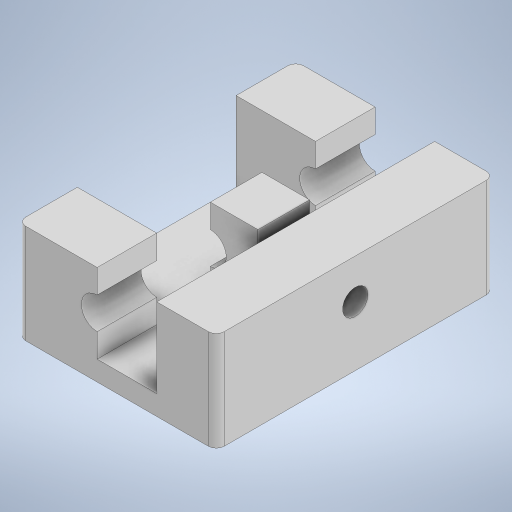
# Autodesk Inventor part: RodBender
Saved by Autodesk Inventor 2023 (Build 270158000, 158)
## iProperties
Created: 2024-04-01
Part Number: RodBender
Material: Generic
Document SubType Name: Modeling
Designer: incep
Density: 1 g/cm^3
Appearance: Default
Author: incep
## iProperties of the stored document RodBender_3DPrint.ipt
Created: 2024-04-01
Part Number: RodBender_3DPrint
Material: Generic
Document SubType Name: Modeling
Designer: incep
Density: 1 g/cm^3
Appearance: Default
Author: incep
Autodesk Inventor part; units mm, degrees
ref_plane "YZ Plane" through (0, 0, 0) normal (1, 0, 0) x (0, 1, 0)
ref_plane "XZ Plane" through (0, 0, 0) normal (0, 1, 0) x (-1, 0, 0)
ref_plane "XY Plane" through (0, 0, 0) normal (0, 0, 1) x (1, 0, 0)
sketch "Sketch1" plane through (0, 0, 0) normal (0, 1, 0) x (-1, 0, 0)
  line L0 (25, -35) -> (-25, -35)
  line L1 (-25, -35) -> (-25, 35)
  line L2 (-25, 35) -> (25, 35)
  line L3 (25, 35) -> (25, -35)
  line L4 (25, -35) -> (5, -35)
  line L5 (5, -35) -> (5, 35)
  line L6 (5, 35) -> (25, 35)
  line L7 (25, 35) -> (25, -35)
  line L8 (-10, -35) -> (-25, -35)
  line L9 (-25, -35) -> (-25, 35)
  line L10 (-25, 35) -> (-10, 35)
  line L11 (-10, 35) -> (-10, -35)
  line L12 (5, 6.5) -> (-7, 6.5)
  line L13 (-7, 6.5) -> (-7, -6.5)
  line L14 (-7, -6.5) -> (5, -6.5)
  line L15 (5, -6.5) -> (5, 6.5)
  point P0 (0, 0)
  point P1 (-25, 0)
  point P2 (0, -35)
  point P3 (5, 0)
  point P4 (5, -35)
  point P5 (-10, -7.5)
  point P6 (5, -6.5)
  point P7 (5, 6.5)
  point P8 (-10, 7.5)
  dimension "d0" = 70
  dimension "d1" = 50
  dimension "d2" = 20
  dimension "d3" = 15
  dimension "d4" = 13
  dimension "d16" = 3
  constraints: 32 end point, 8 parallel, 4 horizontal, 4 midpoint, 4 perpendicular, 2 point on line, 1 collinear, 1 horizontal alignment, 1 vertical alignment
  measures "d0" distance of L2.end L0.start
  measures "d1" distance of L0.start L0.end
  measures "d2" distance between parallel lines of L5 L3
  measures "d3" distance between parallel lines of L1 L11
  measures "d4" distance between parallel lines of L14 L12
  measures "d16" distance between parallel lines of L11 L13
extrude "Extrusion1" add sketch "Sketch1" against normal blind 5
extrude "Extrusion2" add sketch "Sketch1" along normal blind 20 contours L0 L5 L2 L3 | L0 L1 L2 L11
extrude "Extrusion3" add sketch "Sketch1" along normal blind 20 separate body contours L14 L13 L12 L5
sketch "Sketch2" plane through (25, -5, -35) normal (0, 0, -1) x (-1, 0, 0)
  line L0 (30, 5) -> (30, 25) projected
  circle A0 centre (30, 15) radius 4
  point P0 (25, 5)
  dimension "d11" = 8
  constraints: 1 centre point, 1 midpoint
  measures "d11" diameter of A0
extrude "Extrusion4" cut sketch "Sketch2" against normal up to surface (70 mm away) bodies 1
extrude "Extrusion5" cut sketch "Sketch2" against normal up to surface (70 mm away) bodies 2
sketch "Sketch3" plane through (0, 20, 0) normal (0, 1, 0) x (1, 0, 0)
  line L0 (-25, -35) -> (-25, 35) projected
  line L1 (-5, -35) -> (-5, 35) projected
  line L2 (-25, 20) -> (-5, 20)
  line L3 (-5, 20) -> (-5, -20)
  line L4 (-5, -20) -> (-25, -20)
  line L5 (-25, -20) -> (-25, 20)
  point P0 (0, 0)
  point P1 (-25, 0)
  point P2 (-5, 20)
  dimension "d17" = 40
  constraints: 8 end point, 2 midpoint, 2 parallel, 2 point on line, 1 horizontal, 1 perpendicular
  measures "d17" distance between parallel lines of L4 L2
extrude "Extrusion6" cut sketch "Sketch3" against normal up to surface (20 mm away) bodies 1
sketch "Sketch4" plane through (25, -5, 35) normal (1, 0, 0) x (0, 0, -1)
  line L0 (35, 5) -> (35, 25) construction
  line L1 (28.5, 25) -> (41.5, 25) construction
  circle A0 centre (35, 15) radius 3.2
  dimension "d20" = 6.4
  constraints: 2 end point, 2 midpoint, 1 centre point
  measures "d20" diameter of A0
extrude "Extrusion7" cut sketch "Sketch4" against normal up to surface (15 mm away) bodies 1
fillet "Fillet1" radius 2 4 edges at (-25, 7.5, 35) (25, 7.5, 35) (-25, 7.5, -35) (25, 7.5, -35)
body "Solid1"
body "Solid2"
